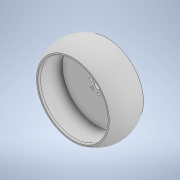
# Autodesk Inventor part: front wheel
Saved by Autodesk Inventor 2020 (Build 240168000, 168)
## iProperties
Created: 2020-01-04
Part Number: front wheel
Material: Generic
Document SubType Name: Modeling
Designer: my
Density: 1 g/cm^3
Appearance: Default
Author: my
Autodesk Inventor part; units mm, degrees
ref_plane "YZ Plane" through (0, 0, 0) normal (1, 0, 0) x (0, 1, 0)
ref_plane "XZ Plane" through (0, 0, 0) normal (0, 1, 0) x (-1, 0, 0)
ref_plane "XY Plane" through (0, 0, 0) normal (0, 0, 1) x (1, 0, 0)
sketch "Sketch1" plane through (0, 0, 0) normal (0, 0, 1) x (1, 0, 0)
  circle A0 centre (0, 0) radius 37.5
  dimension "d0" = 75
  constraints: 1 centre point, 1 coincident
  measures "d0" diameter of A0
sketch "Sketch2" plane through (0, 0, 0) normal (0, 1, 0) x (-1, 0, 0)
  circle A0 centre (-12, 0) radius 25
  line L0 (-32, -15) -> (0, -15)
  line L1 (0, -15) -> (0, 15)
  line L2 (0, 15) -> (-32, 15)
  line L3 (-32, 15) -> (-32, -15)
  point P0 (0, 0)
  dimension "d1" = 50
  dimension "d2" = 12
  dimension "d3" = 30
  dimension "d4" = 15
  constraints: 8 end point, 2 parallel, 2 point on circle, 1 centre point, 1 horizontal, 1 midpoint, 1 perpendicular
  measures "d1" diameter of A0
  measures "d2" distance of point (0, 0) A0.centre
  measures "d3" distance of L2.end L0.start
  measures "d4" distance from line of point (0, 0) L2
sweep "Sweep1" add profiles "Sketch2" path "Sketch1" contours L3 A0 | L2 L1 L0 L3
shell "Shell1" thickness 2.5 removed faces 1 at (15.987, -0.6443, 15)
sketch "Sketch4" plane through (0, 0, -15) normal (0, 0, -1) x (-1, 0, 0)
  circle A0 centre (1.1928, 5.8802) radius 1.2295 projected
  circle A1 centre (0, 0) radius 2 projected
  circle A2 centre (-1.1928, -5.8802) radius 1.2295 projected
  circle A3 centre (-5.6888, -1.9071) radius 1.2295 projected
  circle A4 centre (-4.496, 3.9731) radius 1.2295 projected
  circle A5 centre (1.1928, 5.8802) radius 1.2295 projected
  circle A6 centre (5.6888, 1.9071) radius 1.2295 projected
  circle A7 centre (4.496, -3.9731) radius 1.2295 projected
  arc A8 (-9.2706, -10.4907) -> (10.4907, -9.2706) centre (0, 0) ccw projected
  arc A9 (10.4907, -9.2706) -> (9.2706, 10.4907) centre (0, 0) ccw projected
  arc A10 (9.2706, 10.4907) -> (-10.4907, 9.2706) centre (0, 0) ccw projected
  arc A11 (-10.4907, 9.2706) -> (-9.2706, -10.4907) centre (0, 0) ccw projected
  point P0 (0, 0)
extrude "Extrusion1" cut sketch "Sketch4" against normal blind 10 contours A0 | A2 | A3 | A4 | A6 | A7
sketch "Sketch6" plane through (0, 0, -15) normal (0, 0, -1) x (-1, 0, 0)
  circle A0 centre (0, 0) radius 2.5
  dimension "d10" = 5
  constraints: 1 centre point, 1 coincident
  measures "d10" diameter of A0
extrude "Extrusion2" cut sketch "Sketch6" against normal blind 10
sketch "Sketch7" plane through (0, 0, -12.5) normal (0, 0, 1) x (1, 0, 0)
  circle A0 centre (0, 0) radius 2.5 projected
  circle A1 centre (5.6888, -1.9071) radius 1.2295 projected
  circle A2 centre (-5.6888, 1.9071) radius 1.2295 projected
  circle A3 centre (4.496, 3.9731) radius 1.2295 projected
  circle A4 centre (1.1928, -5.8802) radius 1.2295 projected
  circle A5 centre (-4.496, -3.9731) radius 1.2295 projected
  circle A6 centre (-1.1928, 5.8802) radius 1.2295 projected
  circle A7 centre (0, 0) radius 30.7083 projected
extrude "Extrusion3" add sketch "Sketch7" along normal blind 6
fillet "Fillet1" radius 1 1 edges at (-28.7705, -0.001, 15)
body "Solid1"
